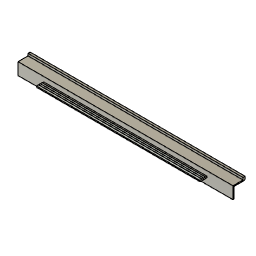
Hafele Handle 126.35.945 (Autodesk Fusion 360 design; units mm, degrees)
description: Handle profile
part number: Hafele 126.35.945
Autodesk Fusion 360 part; units mm, degrees
sketch "Facade" plane through (0, 0, 0) normal (0, 0, 1) x (1, 0, 0)
  line L0 (150, -200) -> (-150, -200)
  line L1 (-150, -200) -> (-150, 200)
  line L2 (-150, 200) -> (150, 200)
  line L3 (150, 200) -> (150, -200)
  line L4 (150, -200) -> (-150, 200) construction
  line L5 (-150, -200) -> (150, 200) construction
  dimension "d4" = 400
  dimension "d5" = 300
  constraint horizontal L0
  constraint perpendicular L0 L1
  constraint parallel L0 L2
  constraint parallel L1 L3
  constraint coincident L4 origin
  constraint coincident L5 origin
  measures "d4" distance of L0.end L1.end
  measures "d5" distance of L1.end L2.end
sketch "Sketch2" plane through (0, 0, 0) normal (1, 0, 0) x (0, 1, 0)
  line L0 (199.9, 0) -> (199.9, -4.5)
  line L1 (199.9, -4.5) -> (184.4, -4.5)
  line L2 (184.4, -4.5) -> (184.4, -19.8)
  line L3 (184.4, -19.8) -> (182.9, -19.8)
  line L4 (182.9, -19.8) -> (182.9, -3)
  line L5 (182.9, -3) -> (196.9, -3)
  line L6 (196.9, -3) -> (196.9, 0)
  line L7 (199.9, 0) -> (196.9, 0)
  point P0 (200, 0)
  dimension "Gap" = 0.1
  dimension "d7" = 3
  dimension "d8" = 1.5
  dimension "d9" = 14
  dimension "d10" = 19.8
  dimension "d11" = 3
  dimension "d13" = 1.5
  constraint vertical L0
  constraint perpendicular L0 L1
  constraint perpendicular L1 L2
  constraint perpendicular L2 L3
  constraint perpendicular L3 L4
  constraint perpendicular L2 L5
  constraint perpendicular L5 L6
  constraint perpendicular L6 L7
  constraint horizontal P0 L0.start
  measures "Gap" distance of P0 L0.start
  measures "d7" distance of L5 L7
  measures "d8" distance of L1 L5
  measures "d9" distance of L4 L6
  measures "d10" distance of P0 L3
  measures "d11" distance of L0 L6
  measures "d13" distance of L2 L4
extrude "Extrude1" add sketch "Sketch2" along normal mid plane 300 makes body 1
sketch "Sketch4" plane through (0, 0, 0) normal (1, 0, 0) x (0, 1, 0)
  line L0 (188.9002, -10.3) -> (164.1797, -10.3)
  line L1 (184.4, -19.8) -> (182.9, -19.8)
  line L2 (182.9, -11.05) -> (180.4, -11.05)
  line L3 (180.4, -11.05) -> (180.4, -11.625)
  line L4 (180.4, -11.625) -> (177.9, -11.05)
  line L5 (177.9, -11.05) -> (177.9, -11.625)
  line L6 (177.9, -11.625) -> (175.4, -11.05)
  line L7 (175.4, -11.05) -> (175.4, -11.625)
  line L8 (175.4, -11.625) -> (172.9, -11.05)
  line L9 (172.9, -11.05) -> (172.9, -10.3)
  line L10 (180.4, -9.55) -> (180.4, -8.975)
  line L11 (175.4, -8.975) -> (172.9, -9.55)
  line L12 (177.9, -9.55) -> (177.9, -8.975)
  line L13 (180.4, -8.975) -> (177.9, -9.55)
  line L14 (175.4, -9.55) -> (175.4, -8.975)
  line L15 (182.9, -9.55) -> (180.4, -9.55)
  line L16 (177.9, -8.975) -> (175.4, -9.55)
  line L17 (172.9, -9.55) -> (172.9, -10.3)
  line L18 (182.9, -19.8) -> (182.9, -3)
  dimension "d26" = 9.5
  dimension "d27" = 1.5
  dimension "d28" = 2.65
  dimension "d29" = 2.5
  dimension "d30" = 2.5
  constraint horizontal L0
  constraint parallel L0 L2
  constraint perpendicular L0 L3
  constraint perpendicular L0 L5
  constraint parallel L4 L6
  constraint parallel L5 L7
  constraint parallel L6 L8
  constraint coincident L0 L9.end
  constraint perpendicular L0 L9
  constraint symmetric L0 L2.start L15.start
  constraint symmetric L0 L2.end L10.start
  constraint symmetric L0 L3.end L10.end
  constraint symmetric L0 L4.end L12.start
  constraint symmetric L0 L5.end L12.end
  constraint symmetric L0 L6.end L14.start
  constraint symmetric L0 L7.end L11.start
  constraint symmetric L0 L8.end L11.end
  constraint symmetric L0 L9.end L17.end
  constraint coincident L2.start L18
  constraint horizontal L3.end L5.end
  constraint horizontal L5.end L7.end
  constraint horizontal L2.end L4.end
  constraint horizontal L4.end L6.end
  constraint horizontal L6.end L8.end
  measures "d26" distance of L0 L1
  measures "d27" distance of L2 L15
  measures "d28" distance of L3.end L10.end
  measures "d29" distance of L2.start L3
  measures "d30" distance of L3 L5
extrude "Extrude2" add sketch "Sketch4" along normal mid plane 228 bodies 1
fillet "Fillet1" radius 2 1 edges at (0, 199.9, -4.5) on bodies 1
sketch "Sketch5" plane through (0, 0, 0) normal (1, 0, 0) x (0, 1, 0)
  line L0 (200, -19) -> (182.9, -19)
  line L1 (182.9, -19) -> (182.9, -3)
  line L2 (182.9, -3) -> (200, -3)
  line L3 (200, -3) -> (200, -19)
  line L4 (182.9, -19.8) -> (182.9, -3)
  line L5 (182.9, -3) -> (196.9, -3)
  line L6 (-200, 0) -> (200, 0)
  line L7 (200, -3) -> (196.9, -3)
  line L8 (196.9, -3) -> (196.9, 0)
  line L9 (196.9, 0) -> (200, 0)
  line L10 (200, 0) -> (200, -3)
  line L11 (196.9, -3) -> (196.9, 0)
  point P0 (200, 0)
  dimension "FacadeThickness" = 19
  constraint horizontal L0
  constraint vertical L1
  constraint horizontal L2
  constraint vertical L3
  constraint vertical L2.end P0
  constraint collinear L1 L4
  constraint collinear L2 L5
  constraint horizontal L7
  constraint vertical L8
  constraint horizontal L9
  constraint vertical L10
  constraint coincident L6 P0
  constraint collinear L8 L11
  measures "FacadeThickness" distance of L0 L6
extrude "Extrude3" add sketch "Sketch5" along normal mid plane 300 separate body makes body 2
sketch "Sketch6" plane through (0, 0, 0) normal (1, 0, 0) x (0, 1, 0)
  line L0 (171.9, -9.3) -> (182.9, -9.3)
  line L1 (182.9, -9.3) -> (182.9, -11.3)
  line L2 (182.9, -11.3) -> (171.9, -11.3)
  line L3 (171.9, -11.3) -> (171.9, -9.3)
  line L4 (171.9, -9.3) -> (182.9, -11.3) construction
  line L5 (182.9, -9.3) -> (171.9, -11.3) construction
  line L6 (172.9, -11.05) -> (172.9, -9.55)
  line L7 (182.9, -19) -> (182.9, -3)
  point P0 (177.4, -10.3)
  point P1 (172.9, -10.3)
  dimension "d39" = 2
  dimension "d40" = 1
  constraint horizontal L0
  constraint perpendicular L0 L1
  constraint parallel L0 L2
  constraint parallel L1 L3
  constraint coincident L4 P0
  constraint coincident L5 P0
  constraint collinear L1 L7
  constraint midpoint L6 P1
  constraint horizontal P0 P1
  measures "d39" distance of L0.start L2.end
  measures "d40" distance of L3 L6.end
extrude "Extrude4" add sketch "Sketch6" along normal mid plane 298 bodies 2
extrude "Extrude5" add 1 faces at (-150, 193.2667, -13.6667) along direction (-1, 0, 0) blind 0.01 on bodies 2 bodies 2
extrude "Extrude6" add 1 faces at (150, 193.2667, -13.6667) along direction (1, 0, 0) blind 0.01 on bodies 2 bodies 2
hidden bodies 2
equation "FacadeWidth = 300 mm"
equation "FacadeHeight = 400 mm"
equation "Shortening = 36 mm"
equation "d4 = FacadeHeight"
equation "d5 = FacadeWidth"
equation "Gap = 0.1 mm" comment "If gap is needed, please enter 20 mm"
equation "d8 = Thickness"
equation "Thickness = 1.5 mm"
equation "d13 = Thickness"
equation "d24 = FacadeWidth"
equation "d30 = d29"
equation "d31 = FacadeWidth - Shortening * 2"
equation "d37 = FacadeWidth"
equation "d41 = FacadeWidth - 2 mm"
named bodies: "Handle", "Cut Body 1"
